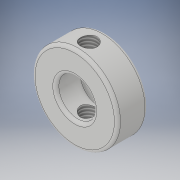
# Autodesk Inventor part: опора
Saved by Autodesk Inventor 2019 (Build 230136000, 136)
## iProperties
Created: 2019-04-29
Part Number: опора
Material: Типовые
Document SubType Name: Modeling
Designer: BarmanKaktus
Density: 1 g/cm^3
Appearance: По умолчанию
Author: BarmanKaktus
Autodesk Inventor part; units mm, degrees
ref_plane "YZ Plane" through (0, 0, 0) normal (1, 0, 0) x (0, 1, 0)
sketch "Эскиз1" plane through (0, 0, 0) normal (0, 0, 1) x (1, 0, 0)
  circle A0 centre (0, 0) radius 7
  dimension "d0" = 14
  constraints: 1 centre point, 1 coincident
  measures "d0" diameter of A0
extrude "Выдавливание1" add sketch "Эскиз1" along normal blind 5
fillet "Сопряжение1" radius 0.5 2 edges at (-7, 0, 5) (-7, 0, 0)
ref_plane "РабПлоскость1" through (0, 0, 5) normal (0, 0, 1) x (1, 0, 0)
sketch "Эскиз2" plane through (0, 0, 5) normal (0, 0, 1) x (1, 0, 0)
  circle A0 centre (0, 0) radius 3.1
  dimension "d5" = 6.2
  constraints: 1 centre point, 1 coincident
  measures "d5" diameter of A0
extrude "Выдавливание2" cut sketch "Эскиз2" against normal blind 4
fillet "Сопряжение2" radius 0.5 1 edges at (-3.1, 0, 5)
ref_plane "РабПлоскость2" through (0, 7, 0) normal (0, 1, 0) x (-1, 0, 0)
sketch "Эскиз3" plane through (0, 7, 0) normal (0, 1, 0) x (-1, 0, 0)
  circle A0 centre (0, 2.7) radius 1.35
  point P0 (0, 0)
  dimension "d10" = 2.7
  dimension "d11" = 2.7
  constraints: 1 centre point
  measures "d10" diameter of A0
  measures "d11" distance of point (0, 0) A0.centre
extrude "Выдавливание3" cut sketch "Эскиз3" against normal through all
thread "Резьба1" size "M3x0.5" class "6H" standard "ANSI Metric M Profile" full length
thread "Резьба2" size "M3x0.5" class "6H" standard "ANSI Metric M Profile" full length
